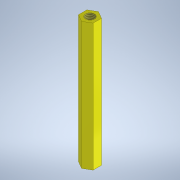
# Autodesk Inventor part: 六角长螺母
Saved by Autodesk Inventor 2020 (Build 240168000, 168)
## iProperties
Part Number: 六角长螺母
Material: 常规
Document SubType Name: Modeling
Designer: YUMEI-design
Mass: 1.78953 g
Surface Area: 22.4262 cm^2
Volume: 1.78953 cm^3
Density: 1 g/cm^3
Appearance: 黄色
Author: YUMEI-design
Autodesk Inventor part; units mm, degrees
ref_plane "YZ Plane" through (0, 0, 0) normal (1, 0, 0) x (0, 1, 0)
ref_plane "XZ Plane" through (0, 0, 0) normal (0, 1, 0) x (-1, 0, 0)
ref_plane "XY Plane" through (0, 0, 0) normal (0, 0, 1) x (1, 0, 0)
sketch "草图1" plane through (0, 0, 0) normal (0, 0, 1) x (1, 0, 0)
  line L0 (0, 4.6188) -> (4, 2.3094)
  line L1 (4, 2.3094) -> (4, -2.3094)
  line L2 (4, -2.3094) -> (0, -4.6188)
  line L3 (0, -4.6188) -> (-4, -2.3094)
  line L4 (-4, -2.3094) -> (-4, 2.3094)
  line L5 (-4, 2.3094) -> (0, 4.6188)
  point P0 (0, 0)
  point P1 (0, 0)
  dimension "d0" = 8
  constraints: 12 end point, 1 coincident, 1 vertical, 13 other
  measures "d0" distance between parallel lines of L1 L4
extrude "拉伸1" add sketch "草图1" along normal mid plane 70
sketch "草图2" plane through (0, 0, 35) normal (0, 0, 1) x (1, 0, 0)
  circle A0 centre (0, 0) radius 2.5
  dimension "d3" = 5
  constraints: 1 centre point, 1 coincident
  measures "d3" diameter of A0
extrude "拉伸2" cut sketch "草图2" against normal through all
thread "螺纹1" size "M5x0.8" class "6H" standard "ANSI Metric M Profile" full length
